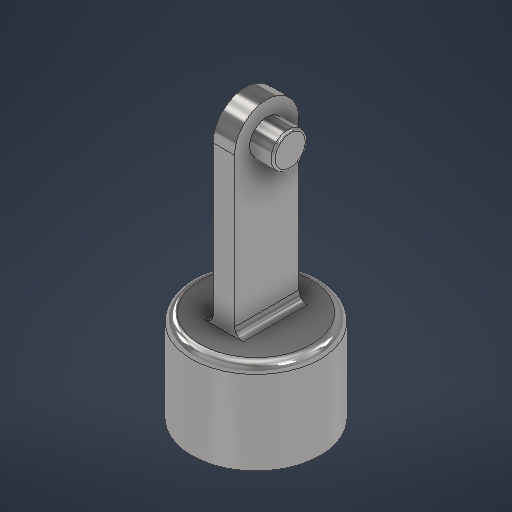
# Autodesk Inventor part: Corpo do robo
Saved by Autodesk Inventor 2026.4 (Build 304435000, 435)
## iProperties
Created: 2026-08-27
Part Number: Corpo do robo
Material: Genérico
Document SubType Name: Modeling
Designer: Matheus
Density: 1 g/cm^3
Appearance: Aço - Polido
Author: Matheus
Autodesk Inventor part; units mm, degrees
ref_plane "YZ Plane" through (0, 0, 0) normal (1, 0, 0) x (0, 1, 0)
ref_plane "XZ Plane" through (0, 0, 0) normal (0, 1, 0) x (-1, 0, 0)
ref_plane "XY Plane" through (0, 0, 0) normal (0, 0, 1) x (1, 0, 0)
sketch "Esboço1" plane through (0, 0, 0) normal (0, 1, 0) x (-1, 0, 0)
  circle A0 centre (0, 0) radius 15
  dimension "d0" = 30
  constraints: 1 centre point, 1 coincident
  measures "d0" diameter of A0
extrude "Extrusão1" add sketch "Esboço1" along normal mid plane 21.5
fillet "Arredondamento1" radius 2 1 edges at (15, 10.75, 0)
sketch "Esboço2" plane through (0, -10.75, 0) normal (0, -1, 0) x (1, 0, 0)
  circle A0 centre (0, 0) radius 5
  dimension "d4" = 10
  constraints: 1 centre point, 1 coincident
  measures "d4" diameter of A0
extrude "Extrusão2" cut sketch "Esboço2" against normal blind 10
sketch "Esboço3" plane through (0, 10.75, 0) normal (0, 1, 0) x (1, 0, 0)
  line L0 (2.5, -7.5) -> (-2.5, -7.5)
  line L1 (-2.5, -7.5) -> (-2.5, 7.5)
  line L2 (-2.5, 7.5) -> (2.5, 7.5)
  line L3 (2.5, 7.5) -> (2.5, -7.5)
  line L4 (2.5, -7.5) -> (-2.5, 7.5) construction
  line L5 (-2.5, -7.5) -> (2.5, 7.5) construction
  point P0 (0, 0)
  dimension "d7" = 5
  dimension "d8" = 15
  constraints: 12 end point, 2 midpoint, 2 parallel, 1 horizontal, 1 perpendicular
  measures "d7" distance between parallel lines of L3 L1
  measures "d8" distance of L0.end L1.end
extrude "Extrusão3" add sketch "Esboço3" along normal blind 44.25
fillet "Arredondamento2" radius 7.5 1 edges at (0, 55, 7.5)
fillet "Arredondamento3" radius 7.5 1 edges at (0, 55, -7.5)
fillet "Arredondamento4" radius 2 1 edges at (2.5, 10.75, 0)
fillet "Arredondamento5" radius 2 1 edges at (-2.5, 10.75, 0)
sketch "Esboço4" plane through (2.5, 47.5, 0) normal (1, 0, 0) x (0, 0, -1)
  line L0 (-7.5, -34.75) -> (-7.5, 0) projected
  line L1 (7.5, -34.75) -> (7.5, 0) projected
  line L2 (-7.5, 0) -> (7.5, 0) construction
  circle A0 centre (0, 0) radius 4
  point P0 (0, -47.5)
  dimension "d15" = 8
  constraints: 2 end point, 1 centre point, 1 horizontal, 1 midpoint
  measures "d15" diameter of A0
extrude "Extrusão4" add sketch "Esboço4" along normal blind 5.5
fillet "Arredondamento6" radius 0.5 1 edges at (8, 47.5, 4)
